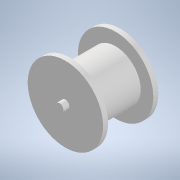
# Autodesk Inventor part: Drum
Saved by Autodesk Inventor 2020 (Build 240168000, 168)
## iProperties
Created: 2020-05-15
Part Number: Drum
Material: Generic
Document SubType Name: Modeling
Designer: jurre
Density: 1 g/cm^3
Appearance: Default
Author: jurre
Autodesk Inventor part; units mm, degrees
ref_plane "YZ Plane" through (0, 0, 0) normal (1, 0, 0) x (0, 1, 0)
ref_plane "XZ Plane" through (0, 0, 0) normal (0, 1, 0) x (-1, 0, 0)
ref_plane "XY Plane" through (0, 0, 0) normal (0, 0, 1) x (1, 0, 0)
sketch "Sketch1" plane through (0, 0, 0) normal (0, 0, 1) x (1, 0, 0)
  arc A0 (2.6458, -2.5) -> (-2.6458, -2.5) centre (0, 0.5) ccw projected
  line L0 (-2.6458, -2.5) -> (2.6458, -2.5) projected
  arc A1 (-2.8983, -2.4) -> (2.8983, -2.4) centre (0, 0.5) ccw
  line L1 (-2.8983, -2.4) -> (2.8983, -2.4)
  circle A2 centre (0, 0.5) radius 11 projected
  circle A3 centre (0, 0.5) radius 18 projected
  circle A4 centre (0, 0.5) radius 18.1
  circle A5 centre (0, 0) radius 25
  circle A6 centre (0, 0) radius 37.5
  dimension "d0" = 0.1
  dimension "d1" = 0.1
  dimension "d2" = 50
  dimension "d3" = 75
  constraints: 4 centre point, 2 coincident, 2 end point, 2 point on circle, 1 other
  measures "d0" radial gap between concentric circles of A0 A1
  measures "d1" radial gap between concentric circles of A3 A4
  measures "d2" diameter of A5
  measures "d3" diameter of A6
extrude "Extrusion1" add sketch "Sketch1" against normal blind 15 contours L1 A0 | A2
sketch "Sketch3" plane through (0, 0.5, 0) normal (0, 0, 1) x (1, 0, 0)
  circle A0 centre (0, 0) radius 11 projected
  circle A1 centre (0, 0) radius 18 projected
  point P0 (0, -0.5)
extrude "Extrusion2" add sketch "Sketch3" against normal blind 19
sketch "Sketch4" plane through (0, 0.5, 0) normal (0, 0, 1) x (1, 0, 0)
  circle A0 centre (0, 0) radius 18 projected
  circle A1 centre (0, 0) radius 25
  point P0 (0, -0.5)
  dimension "d8" = 50
  constraints: 1 centre point, 1 coincident
  measures "d8" diameter of A1
extrude "Extrusion3" add sketch "Sketch4" against normal blind 45
sketch "Sketch5" plane through (0, 0.5, 0) normal (0, 0, 1) x (1, 0, 0)
  circle A0 centre (0, 0) radius 37.5
  point P0 (0, -0.5)
  dimension "d11" = 75
  constraints: 1 centre point
  measures "d11" diameter of A0
extrude "Extrusion4" add sketch "Sketch5" along normal blind 5
sketch "Sketch6" plane through (0, 0.5, -45) normal (0, 0, -1) x (-1, 0, 0)
  circle A0 centre (0, 0) radius 37.5
  circle A1 centre (0, 0) radius 18 projected
  point P0 (0, -0.5)
  dimension "d14" = 75
  constraints: 1 centre point
  measures "d14" diameter of A0
extrude "Extrusion6" add sketch "Sketch6" along normal blind 5
sketch "Sketch8" plane through (0, 0.5, 5) normal (0, 0, 1) x (1, 0, 0)
  arc A0 (2.6458, -3) -> (-2.6458, -3) centre (0, 0) ccw projected
  line L0 (-2.6458, -3) -> (2.6458, -3) projected
  circle A1 centre (0, 0) radius 4
  point P0 (0, -0.5)
  point P1 (4, 0)
  point P2 (2.6458, -3)
  constraints: 1 centre point, 1 coincident, 1 concentric
extrude "Extrusion7" add sketch "Sketch8" along normal blind 6
body "Solid1"
